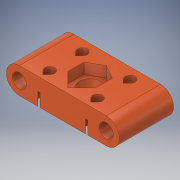
# Autodesk Inventor part: Hopper Nut Trap
Saved by Autodesk Inventor 2018 (Build 220112000, 112)
## iProperties
Created: 2013-10-19
Part Number: Hopper Nut Trap
Material: ABS Plastic
Document SubType Name: Modeling
Designer: Gabriel Smolnycki
Mass: 10.5479 g
Surface Area: 61.8833 cm^2
Volume: 9.95086 cm^3
Density: 1.06 g/cm^3
Appearance: Smooth - Light Orange
Sending System: SolidWorks 2017
Last Author: Gabriel Smolnycki
Last Saved: 2017-09-14
Author: Gabriel Smolnycki
Autodesk Inventor part; units mm, degrees
ref_plane "YZ Plane" through (0, 0, 0) normal (1, 0, 0) x (0, 1, 0)
ref_plane "XZ Plane" through (0, 0, 0) normal (0, 1, 0) x (-1, 0, 0)
ref_plane "Work Plane1" through (0, 0, -12.5) normal (0, 0, 1) x (1, 0, 0)
sketch "Sketch1" plane through (0, 0, -12.5) normal (0, 0, 1) x (1, 0, 0)
  arc A0 (20, -6) -> (20, 6) centre (20, 0) ccw
  line L0 (20, 6) -> (-20, 6)
  arc A1 (-20, 6) -> (-20, -6) centre (-20, 0) ccw
  line L1 (-20, -6) -> (20, -6)
  constraints: 4 end point, 4 point on circle, 2 centre point, 2 horizontal, 1 equal radius, 1 parallel
extrude "Extrusion12" add sketch "Sketch1" along normal blind 25
sketch "Sketch2" plane through (-20, -6, -12.5) normal (0, -1, 0) x (1, 0, 0)
  line L0 (31, 10.5207) -> (27.5, 7.0207)
  line L1 (34.5, 7.0207) -> (31, 10.5207)
  line L2 (34.5, 2.9793) -> (34.5, 7.0207)
  line L3 (31, 0.9585) -> (34.5, 2.9793)
  line L4 (27.5, 2.9793) -> (31, 0.9585)
  line L5 (27.5, 7.0207) -> (27.5, 2.9793)
  constraints: 12 end point, 4 equal length, 2 vertical, 1 perpendicular
extrude "Extrusion11" cut sketch "Sketch2" against normal blind 6 draft 0
sketch "Sketch3" plane through (-20, -6, -12.5) normal (0, -1, 0) x (1, 0, 0)
  line L0 (9, 10.5207) -> (5.5, 7.0207)
  line L1 (12.5, 7.0207) -> (9, 10.5207)
  line L2 (12.5, 2.9793) -> (12.5, 7.0207)
  line L3 (9, 0.9585) -> (12.5, 2.9793)
  line L4 (5.5, 2.9793) -> (9, 0.9585)
  line L5 (5.5, 7.0207) -> (5.5, 2.9793)
  constraints: 12 end point, 4 equal length, 2 vertical, 1 perpendicular
extrude "Extrusion10" cut sketch "Sketch3" against normal blind 6 draft 0
sketch "Sketch4" plane through (-20, -6, -12.5) normal (0, -1, 0) x (1, 0, 0)
  line L0 (5.5, 22.0207) -> (5.5, 17.9793)
  line L1 (8.4793, 25) -> (9.5207, 25)
  line L2 (9, 15.9585) -> (12.5, 17.9793)
  line L3 (8.4793, 25) -> (5.5, 22.0207)
  line L4 (12.5, 22.0207) -> (9.5207, 25)
  line L5 (5.5, 17.9793) -> (9, 15.9585)
  line L6 (12.5, 17.9793) -> (12.5, 22.0207)
  constraints: 14 end point, 4 equal length, 2 vertical, 1 horizontal, 1 perpendicular
extrude "Extrusion9" cut sketch "Sketch4" against normal blind 6 draft 0
sketch "Sketch5" plane through (-20, -6, -12.5) normal (0, -1, 0) x (1, 0, 0)
  line L0 (31, 15.9585) -> (34.5, 17.9793)
  line L1 (30.4793, 25) -> (27.5, 22.0207)
  line L2 (34.5, 22.0207) -> (31.5207, 25)
  line L3 (27.5, 17.9793) -> (31, 15.9585)
  line L4 (31.5207, 25) -> (30.4793, 25)
  line L5 (34.5, 17.9793) -> (34.5, 22.0207)
  line L6 (27.5, 22.0207) -> (27.5, 17.9793)
  constraints: 14 end point, 4 equal length, 2 vertical, 1 horizontal, 1 perpendicular
extrude "Extrusion8" cut sketch "Sketch5" against normal blind 6
sketch "Sketch6" plane through (0, 0, 0) normal (0, 1, 0) x (-1, 0, 0)
  arc A0 (-12.591, 9.091) -> (-9.409, 9.091) centre (-11, 7.5) ccw
  line L0 (-12.591, 9.091) -> (-11, 10.682)
  line L1 (-11, 10.682) -> (-9.409, 9.091)
  constraints: 4 end point, 2 perpendicular, 2 point on circle, 1 centre point
extrude "Extrusion7" cut sketch "Sketch6" along normal blind 6 draft 0
sketch "Sketch7" plane through (-20, 6, -12.5) normal (0, 1, 0) x (1, 0, 0)
  line L0 (7.409, -21.591) -> (9, -23.182)
  arc A0 (10.591, -21.591) -> (7.409, -21.591) centre (9, -20) ccw
  line L1 (9, -23.182) -> (10.591, -21.591)
  constraints: 4 end point, 2 perpendicular, 2 point on circle, 1 centre point
extrude "Extrusion6" cut sketch "Sketch7" against normal blind 6
sketch "Sketch8" plane through (-20, 6, -12.5) normal (0, 1, 0) x (1, 0, 0)
  arc A0 (32.591, -6.591) -> (29.409, -6.591) centre (31, -5) ccw
  line L0 (31, -8.182) -> (32.591, -6.591)
  line L1 (29.409, -6.591) -> (31, -8.182)
  constraints: 4 end point, 2 perpendicular, 2 point on circle, 1 centre point
extrude "Extrusion5" cut sketch "Sketch8" against normal blind 6
sketch "Sketch9" plane through (-20, 6, -12.5) normal (0, 1, 0) x (1, 0, 0)
  arc A0 (10.591, -6.591) -> (7.409, -6.591) centre (9, -5) ccw
  line L0 (9, -8.182) -> (10.591, -6.591)
  line L1 (7.409, -6.591) -> (9, -8.182)
  constraints: 4 end point, 2 perpendicular, 2 point on circle, 1 centre point
extrude "Extrusion4" cut sketch "Sketch9" against normal blind 6
sketch "Sketch10" plane through (-20, 6, -12.5) normal (0, 1, 0) x (1, 0, 0)
  line L0 (20, -22.7528) -> (26.5, -16.2528)
  line L1 (13.5, -16.2528) -> (20, -22.7528)
  line L2 (13.5, -8.7472) -> (13.5, -16.2528)
  line L3 (20, -4.9944) -> (13.5, -8.7472)
  line L4 (26.5, -8.7472) -> (20, -4.9944)
  line L5 (26.5, -16.2528) -> (26.5, -8.7472)
  constraints: 12 end point, 4 equal length, 2 vertical, 1 perpendicular
extrude "Extrusion3" cut sketch "Sketch10" against normal blind 5 draft 0
sketch "Sketch11" plane through (-20, -6, -12.5) normal (0, -1, 0) x (1, 0, 0)
  line L0 (20, 23.8137) -> (14.3431, 18.1569)
  line L1 (25.6569, 18.1569) -> (20, 23.8137)
  arc A0 (14.3431, 18.1569) -> (25.6569, 18.1569) centre (20, 12.5) ccw
  constraints: 4 end point, 2 perpendicular, 2 point on circle, 1 centre point
extrude "Extrusion2" cut sketch "Sketch11" against normal blind 2 draft 0
sketch "Sketch12" plane through (-20, 1, -12.5) normal (0, 1, 0) x (1, 0, 0)
  arc A0 (23.5355, -16.0355) -> (16.4645, -16.0355) centre (20, -12.5) ccw
  line L0 (20, -19.5711) -> (23.5355, -16.0355)
  line L1 (16.4645, -16.0355) -> (20, -19.5711)
  constraints: 4 end point, 2 perpendicular, 2 point on circle, 1 centre point
extrude "Extrusion1" cut sketch "Sketch12" against normal blind 5
hole "Hole2" at (20, 0, 12.5) direction (0, 0, -1) diameter 6.5 depth 25
sketch "Sketch13" plane through (0, 0, 12.5) normal (0, 0, 1) x (1, 0, 0)
  point P0 (20, 0)
hole "Hole1" at (-20, 0, 12.5) direction (0, 0, -1) diameter 6.5 depth 25
sketch "Sketch14" plane through (0, 0, 12.5) normal (0, 0, 1) x (1, 0, 0)
  point P0 (-20, 0)
body "Solid3"
